Rahmen_Schrank_v2 (Autodesk Fusion 360 design; units mm, degrees)
Autodesk Fusion 360 part; units mm, degrees
note: some values were not read from the file. Set by a fixed rule: which sketch regions a step uses; which face or edge a step refers to.
sketch "Skizze1" plane through (0, 0, 0) normal (0, 1, 0) x (1, 0, 0)
  line L0 (0, 0) -> (295, 0)
  line L1 (0, 0) -> (0, -464)
  line L2 (0, -464) -> (295, -464)
  line L3 (295, -464) -> (295, 0)
  line L4 (0, 0) -> (32, 0)
  line L5 (32, 0) -> (32, -10) construction
  line L6 (32, -10) -> (263, -10) construction
  line L7 (32, -15) -> (32, -454)
  line L8 (32, -454) -> (263, -454) construction
  line L9 (263, -454) -> (263, -15)
  line L10 (0, -464) -> (15.5, -464)
  line L11 (15.5, -464) -> (15.5, -348) construction
  line L12 (15.5, -348) -> (15.5, -116) construction
  line L13 (15.5, -116) -> (277.5, -116)
  line L14 (15.5, -348) -> (277.5, -348) construction
  circle A0 centre (15.5, -116) radius 6.5
  line L15 (23.5, -118.5) -> (7.5, -118.5)
  line L16 (7.5, -118.5) -> (7.5, -113.5)
  line L17 (7.5, -113.5) -> (23.5, -113.5)
  line L18 (23.5, -113.5) -> (23.5, -118.5)
  line L19 (23.5, -118.5) -> (7.5, -113.5) construction
  line L20 (7.5, -118.5) -> (23.5, -113.5) construction
  line L21 (285.5, -118.5) -> (269.5, -118.5)
  line L22 (269.5, -118.5) -> (269.5, -113.5)
  line L23 (269.5, -113.5) -> (285.5, -113.5)
  circle A1 centre (277.5, -116) radius 6.5
  line L24 (285.5, -113.5) -> (285.5, -118.5)
  line L25 (23.5, -345.5) -> (23.5, -350.5)
  line L26 (23.5, -350.5) -> (7.5, -345.5) construction
  line L27 (7.5, -345.5) -> (23.5, -345.5)
  circle A2 centre (15.5, -348) radius 6.5
  line L28 (23.5, -350.5) -> (7.5, -350.5)
  line L29 (7.5, -350.5) -> (7.5, -345.5)
  line L30 (7.5, -350.5) -> (23.5, -345.5) construction
  circle A3 centre (277.5, -348) radius 6.5
  line L31 (285.5, -345.5) -> (285.5, -350.5)
  line L32 (269.5, -350.5) -> (269.5, -345.5)
  line L33 (269.5, -345.5) -> (285.5, -345.5)
  line L34 (285.5, -350.5) -> (269.5, -350.5)
  line L35 (32, -15) -> (263, -15)
  line L36 (32, -454) -> (32, -449)
  line L37 (32, -449) -> (263, -449)
  line L38 (0, -464) -> (0, -314)
  line L39 (0, -314) -> (295, -314)
  line L40 (0, 0) -> (0, -150)
  line L41 (0, -150) -> (295, -150)
  line L42 (15.5, -157.494) -> (8.4703, -153.6752) construction
  line L43 (15.5, -157.494) -> (12.6999, -150) construction
  line L44 (15.5, -314) -> (15.5, -264) construction
  line L45 (15.5, -314) -> (15.5, -306.5)
  line L46 (15.5, -306.5) -> (277.5, -306.5) construction
  line L47 (277.5, -306.5) -> (277.5, -157.494)
  arc A4 (18.2839, -314) -> (12.7161, -314) centre (15.5, -306.5) ccw
  arc A5 (18.5594, -314) -> (12.4406, -314) centre (15.5, -306.5) ccw
  arc A6 (280.2839, -314) -> (274.7161, -314) centre (277.5, -306.5) ccw
  arc A7 (280.5594, -314) -> (274.4406, -314) centre (277.5, -306.5) ccw
  arc A8 (274.4258, -150) -> (280.5742, -150) centre (277.5, -157.494) ccw
  arc A9 (274.6999, -150) -> (280.3001, -150) centre (277.5, -157.494) ccw
  arc A10 (12.4258, -150) -> (18.5742, -150) centre (15.5, -157.494) ccw
  arc A11 (8.4703, -153.6752) -> (18.3001, -150) centre (15.5, -157.494) ccw
  arc A12 (12.6999, -150) -> (18.3001, -150) centre (15.5, -157.494) ccw
  line L48 (0, 0) -> (147.5, 0)
  line L49 (147.5, 0) -> (147.5, -15)
  line L50 (147.5, -15) -> (147.5, -449) construction
  line L51 (147.5, -7.5) -> (152.5, -7.5)
  arc A13 (147.489, -10) -> (147.5, -4.9781) centre (152.5, -7.5) ccw
  arc A14 (147.5, -9.7913) -> (147.5, -5.2087) centre (152.5, -7.5) ccw
  line L52 (147.5, -449) -> (147.5, -464)
  arc A15 (147.5, -458.7913) -> (147.5, -454.2087) centre (152.5, -456.5) ccw
  arc A16 (147.489, -459) -> (147.5, -453.9781) centre (152.5, -456.5) ccw
  point P0 (15.5, -116)
  point P1 (15.5, -348)
  point P2 (15.5, -348)
  point P3 (277.5, -348)
  dimension "d1" = 295
  dimension "d2" = 464
  dimension "d3" = 32
  dimension "d4" = 10
  dimension "d5" = 231
  dimension "d6" = 444
  dimension "d7" = 15.5
  dimension "d8" = 116
  dimension "d9" = 232
  dimension "d10" = 262
  dimension "d11" = 262
  dimension "d12" = 13
  dimension "d13" = 16
  dimension "d14" = 5
  dimension "d15" = 13
  dimension "d16" = 16
  dimension "d17" = 5
  dimension "d18" = 13
  dimension "d19" = 16
  dimension "d20" = 5
  dimension "d21" = 13
  dimension "d22" = 16
  dimension "d23" = 5
  dimension "d24" = 5
  dimension "d25" = 5
  dimension "d26" = 150
  dimension "d27" = 150
  dimension "d28" = 16
  dimension "d29" = 16.2
  dimension "d31" = 7.5
  dimension "d32" = 16
  dimension "d33" = 16.2
  dimension "d34" = 16
  dimension "d35" = 16.2
  dimension "d36" = 16
  dimension "d37" = 16.2
  dimension "d38" = 147.5
  dimension "d39" = 5
  dimension "d40" = 11
  dimension "d41" = 11.2
  dimension "d42" = 11
  dimension "d43" = 11.2
  constraint coincident L0.start L1.start
  constraint horizontal L0
  constraint perpendicular L0 L1
  constraint perpendicular L1 L2
  constraint perpendicular L0 L3
  constraint perpendicular L1 L4
  constraint vertical L5
  constraint perpendicular L5 L6
  constraint perpendicular L6 L7
  constraint perpendicular L7 L8
  constraint perpendicular L6 L9
  constraint perpendicular L1 L10
  constraint perpendicular L2 L11
  constraint parallel L11 L12
  constraint perpendicular L9 L13
  constraint perpendicular L9 L14
  constraint coincident P0 L12.end
  constraint horizontal L15
  constraint perpendicular L15 L16
  constraint parallel L15 L17
  constraint parallel L16 L18
  constraint coincident L19 P0
  constraint coincident L20 P0
  constraint horizontal L21
  constraint perpendicular L21 L22
  constraint parallel L21 L23
  constraint parallel L22 L24
  constraint coincident P2 P1
  constraint horizontal L28
  constraint perpendicular L28 L29
  constraint parallel L27 L28
  constraint parallel L25 L29
  constraint coincident P2 L26
  constraint coincident P2 L30
  constraint horizontal L34
  constraint perpendicular L32 L34
  constraint parallel L33 L34
  constraint parallel L31 L32
  constraint perpendicular L9 L35
  constraint perpendicular L2 L36
  constraint coincident L9 L37.end
  constraint perpendicular L9 L37
  constraint perpendicular L2 L38
  constraint coincident L3 L39.end
  constraint perpendicular L3 L39
  constraint perpendicular L0 L40
  constraint coincident L3 L41.end
  constraint perpendicular L3 L41
  constraint coincident L12 L42.start
  constraint concentric A10 A12
  constraint coincident L41 L43.end
  constraint coincident L42.start L43.start
  constraint coincident L12 L44.start
  constraint coincident L39 L44.start
  constraint coincident L12 L44.end
  constraint perpendicular L39 L45
  constraint perpendicular L45 L46
  constraint perpendicular L41 L47
  constraint coincident L45.end L46.start
  constraint concentric A4 A5
  constraint concentric A8 A9
  constraint concentric A6 A7
  constraint coincident L39 A4.start
  constraint coincident L39 A4.end
  constraint coincident L39 A5.end
  constraint coincident L39 A5.start
  constraint coincident L39 A6.end
  constraint coincident L39 A6.start
  constraint coincident L39 A7.end
  constraint coincident L39 A7.start
  constraint coincident L41 A8.end
  constraint coincident L41 A8.start
  constraint coincident L41 A9.end
  constraint coincident L41 A9.start
  constraint coincident L41 A10.end
  constraint coincident L41 A11.end
  constraint coincident L41 A10.start
  constraint perpendicular L40 L48
  constraint midpoint L35 L49.end
  constraint perpendicular L35 L49
  constraint midpoint L37 L50.end
  constraint midpoint L49 L51.start
  constraint perpendicular L49 L51
  constraint coincident L51.end A13.centre
  constraint concentric A13 A14
  constraint coincident L49 A13.end
  constraint coincident L6 A13.start
  constraint coincident L49 A14.end
  constraint coincident L49 A14.start
  constraint concentric A15 A16
  constraint coincident A16.end L52
  constraint coincident A15.end L52
  constraint coincident A15.start L52
  measures "d1" distance of L0.start L0.end
  measures "d2" distance of L0.start L1.end
  measures "d3" distance of L0.start L4.end
  measures "d4" distance of L4.end L5.end
  measures "d5" distance of L5.end L6.end
  measures "d6" distance of L5.end L7.end
  measures "d7" distance of L1.end L10.end
  measures "d8" distance of L10.end P2
  measures "d9" distance of P2 P0
  measures "d10" distance of P0 L13.end
  measures "d11" distance of P2 P3
  measures "d12" diameter of A0
  measures "d13" distance of L16.end L17.end
  measures "d14" distance of L15.end L16.end
  measures "d15" diameter of A1
  measures "d16" distance of L22.end L23.end
  measures "d17" distance of L22.end L21.end
  measures "d18" diameter of A2
  measures "d19" distance of L26.end L25.start
  measures "d20" distance of L26.end L28.end
  measures "d21" diameter of A3
  measures "d22" distance of L31.start L32.end
  measures "d23" distance of L32.start L32.end
  measures "d24" distance of L5.end L7.start
  measures "d25" distance of L7.end L36.end
  measures "d26" distance of L1.end L38.end
  measures "d27" distance of L0.start L40.end
  measures "d28" diameter of A12
  measures "d29" diameter of A10
  measures "d31" distance of L44.start L45.end
  measures "d32" diameter of A4
  measures "d33" diameter of A5
  measures "d34" diameter of A9
  measures "d35" diameter of A8
  measures "d36" diameter of A6
  measures "d37" diameter of A7
  measures "d38" distance of L0.start L48.end
  measures "d39" distance of L51.start L51.end
  measures "d40" diameter of A14
  measures "d41" diameter of A13
  measures "d42" diameter of A15
  measures "d43" diameter of A16
extrude "Extrusion1" add sketch "Skizze1" along normal blind 5 contours L2 L3 L9 L37 L39 L52 A16 | L39 A6 makes body 1
extrude "Extrusion2" add sketch "Skizze1" along normal blind 5 separate body contours L1 L2 L7 L10 L37 L38 L39 L52 | L39 A4 | L52 A15 makes body 2
extrude "Extrusion3" add sketch "Skizze1" along normal blind 5 separate body contours L1 L7 L39 L41 A5 A10 makes body 3
extrude "Extrusion4" add sketch "Skizze1" along normal blind 5 separate body contours L0 L1 L4 L7 L35 L40 L41 L48 L49 | L41 A11 A12 | L49 A14 makes body 4
extrude "Extrusion5" add sketch "Skizze1" along normal blind 5 separate body contours L0 L3 L9 L35 L41 L49 A13 | L41 A9 makes body 5
extrude "Extrusion6" add sketch "Skizze1" along normal blind 5 separate body contours L3 L39 L41 L47 A7 A8 | L9 L39 L41 L47 A7 A8 makes body 6
move_face "Fläche verschieben1" by (0, -2, 0) 6 faces at (291.23, 5, 255.0918) (279.4248, 5, 422.2927) (15.2055, 5, 422.407) (28.7237, 5, 255.3019) (15.2055, 5, 41.593) (279.4248, 5, 41.7073) on bodies 1 2 3 4 5 6
move_face "Flächen versetzen1" offset -0.5 2 faces at (5.1667, 1, 464) (196.6667, 1, 464) on bodies 1 2
move_face "Flächen versetzen2" offset -0.5 2 faces at (70.5, 1, 0) (196.6667, 1, 0) on bodies 4 5
